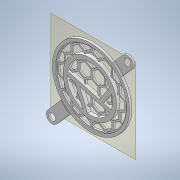
# Autodesk Inventor part: Rear Left Fan Cover
Saved by Autodesk Inventor 2020 (Build 240168000, 168)
## iProperties
Created: 2019-11-19
Part Number: Rear Left Fan Cover
Material: Generic
Document SubType Name: Modeling
Designer: pepd9
Density: 1 g/cm^3
Appearance: Default
Author: pepd9
Autodesk Inventor part; units mm, degrees
ref_plane "YZ Plane" through (0, 0, 0) normal (1, 0, 0) x (0, 1, 0)
ref_plane "XZ Plane" through (0, 0, 0) normal (0, 1, 0) x (-1, 0, 0)
ref_plane "XY Plane" through (0, 0, 0) normal (0, 0, 1) x (1, 0, 0)
sketch "Sketch1" plane through (0, 0, 0) normal (0, 0, 1) x (1, 0, 0)
  circle A0 centre (0, 0) radius 17.5
  circle A1 centre (0, 0) radius 19.5
  dimension "d0" = 35
  dimension "d1" = 2
  constraints: 2 centre point, 1 coincident
  measures "d0" diameter of A0
  measures "d1" radial gap between concentric circles of A0 A1
extrude "Extrusion1" add sketch "Sketch1" along normal blind 0.8
ref_plane "Work Plane1" through (0, 0, 0) normal (0, 0, 1) x (1, 0, 0)
sketch "Sketch2" plane through (0, 0, 0) normal (0, 0, 1) x (1, 0, 0)
  line L0 (0, 3.4641) -> (3, 1.7321)
  line L1 (3, 1.7321) -> (3, -1.7321)
  line L2 (3, -1.7321) -> (0, -3.4641)
  line L3 (0, -3.4641) -> (-3, -1.7321)
  line L4 (-3, -1.7321) -> (-3, 1.7321)
  line L5 (-3, 1.7321) -> (0, 3.4641)
  line L6 (0, 4.3879) -> (3.8, 2.1939)
  line L7 (3.8, 2.1939) -> (3.8, -2.1939)
  line L8 (3.8, -2.1939) -> (0, -4.3879)
  line L9 (0, -4.3879) -> (-3.8, -2.1939)
  line L10 (-3.8, -2.1939) -> (-3.8, 2.1939)
  line L11 (-3.8, 2.1939) -> (0, 4.3879)
  line L12 (26.5453, -9.9641) -> (29.5453, -11.6962)
  line L13 (29.5453, -11.6962) -> (29.5453, -15.1603)
  line L14 (29.5453, -15.1603) -> (26.5453, -16.8923)
  line L15 (26.5453, -16.8923) -> (23.5453, -15.1603)
  line L16 (23.5453, -15.1603) -> (23.5453, -11.6962)
  line L17 (23.5453, -11.6962) -> (26.5453, -9.9641)
  line L18 (26.5453, -9.0403) -> (30.3453, -11.2343)
  line L19 (30.3453, -11.2343) -> (30.3453, -15.6221)
  line L20 (30.3453, -15.6221) -> (26.5453, -17.8161)
  line L21 (26.5453, -17.8161) -> (22.7453, -15.6221)
  line L22 (22.7453, -15.6221) -> (22.7453, -11.2343)
  line L23 (22.7453, -11.2343) -> (26.5453, -9.0403)
  line L24 (-6.8, 3.4641) -> (-3.8, 1.7321)
  line L25 (-3.8, 1.7321) -> (-3.8, -1.7321)
  line L26 (-3.8, -1.7321) -> (-6.8, -3.4641)
  line L27 (-6.8, -3.4641) -> (-9.8, -1.7321)
  line L28 (-9.8, -1.7321) -> (-9.8, 1.7321)
  line L29 (-9.8, 1.7321) -> (-6.8, 3.4641)
  line L30 (-6.8, 4.3879) -> (-3, 2.1939)
  line L31 (-3, 2.1939) -> (-3, -2.1939)
  line L32 (-3, -2.1939) -> (-6.8, -4.3879)
  line L33 (-6.8, -4.3879) -> (-10.6, -2.1939)
  line L34 (-10.6, -2.1939) -> (-10.6, 2.1939)
  line L35 (-10.6, 2.1939) -> (-6.8, 4.3879)
  line L36 (-13.6, 3.4641) -> (-10.6, 1.7321)
  line L37 (-10.6, 1.7321) -> (-10.6, -1.7321)
  line L38 (-10.6, -1.7321) -> (-13.6, -3.4641)
  line L39 (-13.6, -3.4641) -> (-16.6, -1.7321)
  line L40 (-16.6, -1.7321) -> (-16.6, 1.7321)
  line L41 (-16.6, 1.7321) -> (-13.6, 3.4641)
  line L42 (-13.6, 4.3879) -> (-9.8, 2.1939)
  line L43 (-9.8, 2.1939) -> (-9.8, -2.1939)
  line L44 (-9.8, -2.1939) -> (-13.6, -4.3879)
  line L45 (-13.6, -4.3879) -> (-17.4, -2.1939)
  line L46 (-17.4, -2.1939) -> (-17.4, 2.1939)
  line L47 (-17.4, 2.1939) -> (-13.6, 4.3879)
  line L48 (-20.4, 3.4641) -> (-17.4, 1.7321)
  line L49 (-17.4, 1.7321) -> (-17.4, -1.7321)
  line L50 (-17.4, -1.7321) -> (-20.4, -3.4641)
  line L51 (-20.4, -3.4641) -> (-23.4, -1.7321)
  line L52 (-23.4, -1.7321) -> (-23.4, 1.7321)
  line L53 (-23.4, 1.7321) -> (-20.4, 3.4641)
  line L54 (-20.4, 4.3879) -> (-16.6, 2.1939)
  line L55 (-16.6, 2.1939) -> (-16.6, -2.1939)
  line L56 (-16.6, -2.1939) -> (-20.4, -4.3879)
  line L57 (-20.4, -4.3879) -> (-24.2, -2.1939)
  line L58 (-24.2, -2.1939) -> (-24.2, 2.1939)
  line L59 (-24.2, 2.1939) -> (-20.4, 4.3879)
  line L60 (6.8, 3.4641) -> (9.8, 1.7321)
  line L61 (9.8, 1.7321) -> (9.8, -1.7321)
  line L62 (9.8, -1.7321) -> (6.8, -3.4641)
  line L63 (6.8, -3.4641) -> (3.8, -1.7321)
  line L64 (3.8, -1.7321) -> (3.8, 1.7321)
  line L65 (3.8, 1.7321) -> (6.8, 3.4641)
  line L66 (6.8, 4.3879) -> (10.6, 2.1939)
  line L67 (10.6, 2.1939) -> (10.6, -2.1939)
  line L68 (10.6, -2.1939) -> (6.8, -4.3879)
  line L69 (6.8, -4.3879) -> (3, -2.1939)
  line L70 (3, -2.1939) -> (3, 2.1939)
  line L71 (3, 2.1939) -> (6.8, 4.3879)
  line L72 (13.6, 3.4641) -> (16.6, 1.7321)
  line L73 (16.6, 1.7321) -> (16.6, -1.7321)
  line L74 (16.6, -1.7321) -> (13.6, -3.4641)
  line L75 (13.6, -3.4641) -> (10.6, -1.7321)
  line L76 (10.6, -1.7321) -> (10.6, 1.7321)
  line L77 (10.6, 1.7321) -> (13.6, 3.4641)
  line L78 (13.6, 4.3879) -> (17.4, 2.1939)
  line L79 (17.4, 2.1939) -> (17.4, -2.1939)
  line L80 (17.4, -2.1939) -> (13.6, -4.3879)
  line L81 (13.6, -4.3879) -> (9.8, -2.1939)
  line L82 (9.8, -2.1939) -> (9.8, 2.1939)
  line L83 (9.8, 2.1939) -> (13.6, 4.3879)
  line L84 (17.4, -2.1939) -> (17.4, 2.1939)
  line L85 (10.2, 9.3531) -> (13.2, 7.621)
  line L86 (13.2, 7.621) -> (13.2, 4.1569)
  line L87 (7.2, 4.1569) -> (7.2, 7.621)
  line L88 (7.2, 7.621) -> (10.2, 9.3531)
  line L89 (10.2, 10.2768) -> (14, 8.0829)
  line L90 (14, 8.0829) -> (14, 4.1569)
  line L91 (6.4, 4.1569) -> (6.4, 8.0829)
  line L92 (6.4, 8.0829) -> (10.2, 10.2768)
  line L93 (3.4, 9.3531) -> (6.4, 7.621)
  line L94 (0.4, 4.1569) -> (0.4, 7.621)
  line L95 (0.4, 7.621) -> (3.4, 9.3531)
  line L96 (3.4, 10.2768) -> (6.8, 8.3138)
  line L97 (-0.4, 4.1569) -> (-0.4, 8.0829)
  line L98 (-0.4, 8.0829) -> (3.4, 10.2768)
  line L99 (-3.4, 9.3531) -> (-0.4, 7.621)
  line L100 (-6.4, 4.1569) -> (-6.4, 7.621)
  line L101 (-6.4, 7.621) -> (-3.4, 9.3531)
  line L102 (-3.4, 10.2768) -> (0, 8.3138)
  line L103 (-7.2, 4.1569) -> (-7.2, 8.0829)
  line L104 (-7.2, 8.0829) -> (-3.4, 10.2768)
  line L105 (-10.2, 9.3531) -> (-7.2, 7.621)
  line L106 (-13.2, 4.1569) -> (-13.2, 7.621)
  line L107 (-13.2, 7.621) -> (-10.2, 9.3531)
  line L108 (-10.2, 10.2768) -> (-6.8, 8.3138)
  line L109 (-14, 4.1569) -> (-14, 8.0829)
  line L110 (-14, 8.0829) -> (-10.2, 10.2768)
  line L111 (-17, 9.3531) -> (-14, 7.621)
  line L112 (-20, 4.1569) -> (-20, 7.621)
  line L113 (-20, 7.621) -> (-17, 9.3531)
  line L114 (-17, 10.2768) -> (-13.6, 8.3138)
  line L115 (-20.8, 3.695) -> (-20.8, 8.0829)
  line L116 (-20.8, 8.0829) -> (-17, 10.2768)
  line L117 (13.6, 8.3138) -> (17, 10.2768)
  line L118 (14, 7.621) -> (17, 9.3531)
  line L119 (17, 10.2768) -> (20.8, 8.0829)
  line L120 (17, 9.3531) -> (20, 7.621)
  line L121 (13.6, 15.242) -> (16.6, 13.51)
  line L122 (16.6, 13.51) -> (16.6, 10.0459)
  line L123 (10.6, 10.0459) -> (10.6, 13.51)
  line L124 (10.6, 13.51) -> (13.6, 15.242)
  line L125 (13.6, 16.1658) -> (17.4, 13.9719)
  line L126 (17.4, 13.9719) -> (17.4, 9.584)
  line L127 (9.8, 10.0459) -> (9.8, 13.9719)
  line L128 (9.8, 13.9719) -> (13.6, 16.1658)
  line L129 (6.8, 15.242) -> (9.8, 13.51)
  line L130 (3.8, 10.0459) -> (3.8, 13.51)
  line L131 (3.8, 13.51) -> (6.8, 15.242)
  line L132 (6.8, 16.1658) -> (10.6, 13.9719)
  line L133 (3, 10.0459) -> (3, 13.9719)
  line L134 (3, 13.9719) -> (6.8, 16.1658)
  line L135 (0, 15.242) -> (3, 13.51)
  line L136 (-3, 10.0459) -> (-3, 13.51)
  line L137 (-3, 13.51) -> (0, 15.242)
  line L138 (0, 16.1658) -> (3.4, 14.2028)
  line L139 (-3.8, 10.0459) -> (-3.8, 13.9719)
  line L140 (-3.8, 13.9719) -> (0, 16.1658)
  line L141 (-6.8, 15.242) -> (-3.8, 13.51)
  line L142 (-9.8, 10.0459) -> (-9.8, 13.51)
  line L143 (-9.8, 13.51) -> (-6.8, 15.242)
  line L144 (-6.8, 16.1658) -> (-3.4, 14.2028)
  line L145 (-10.6, 10.0459) -> (-10.6, 13.9719)
  line L146 (-10.6, 13.9719) -> (-6.8, 16.1658)
  line L147 (-13.6, 15.242) -> (-10.6, 13.51)
  line L148 (-16.6, 10.0459) -> (-16.6, 13.51)
  line L149 (-16.6, 13.51) -> (-13.6, 15.242)
  line L150 (-13.6, 16.1658) -> (-10.2, 14.2028)
  line L151 (-17.4, 9.584) -> (-17.4, 13.9719)
  line L152 (-17.4, 13.9719) -> (-13.6, 16.1658)
  line L153 (10.2, 21.131) -> (13.2, 19.399)
  line L154 (13.2, 19.399) -> (13.2, 15.9349)
  line L155 (7.2, 15.9349) -> (7.2, 19.399)
  line L156 (7.2, 19.399) -> (10.2, 21.131)
  line L157 (10.2, 22.0548) -> (14, 19.8608)
  line L158 (14, 19.8608) -> (14, 15.473)
  line L159 (6.4, 15.473) -> (6.4, 19.8608)
  line L160 (6.4, 19.8608) -> (10.2, 22.0548)
  line L161 (3.4, 21.131) -> (6.4, 19.399)
  line L162 (0.4, 15.9349) -> (0.4, 19.399)
  line L163 (0.4, 19.399) -> (3.4, 21.131)
  line L164 (3.4, 22.0548) -> (7.2, 19.8608)
  line L165 (-0.4, 15.473) -> (-0.4, 19.8608)
  line L166 (-0.4, 19.8608) -> (3.4, 22.0548)
  line L167 (-3.4, 21.131) -> (-0.4, 19.399)
  line L168 (-6.4, 15.9349) -> (-6.4, 19.399)
  line L169 (-6.4, 19.399) -> (-3.4, 21.131)
  line L170 (-3.4, 22.0548) -> (0.4, 19.8608)
  line L171 (-7.2, 15.473) -> (-7.2, 19.8608)
  line L172 (-7.2, 19.8608) -> (-3.4, 22.0548)
  line L173 (20.4, -7.3901) -> (17.4, -9.1221)
  line L174 (17.4, -9.1221) -> (14.4, -7.3901)
  line L175 (14.4, -7.3901) -> (14.4, -3.926)
  line L176 (21.2, -7.852) -> (17.4, -10.0459)
  line L177 (17.4, -10.0459) -> (13.6, -7.852)
  line L178 (13.6, -7.852) -> (13.6, -3.4641)
  line L179 (13.6, -7.3901) -> (10.2, -9.3531)
  line L180 (10.2, -9.3531) -> (7.2, -7.621)
  line L181 (7.2, -7.621) -> (7.2, -4.1569)
  line L182 (14, -8.0829) -> (10.2, -10.2768)
  line L183 (10.2, -10.2768) -> (6.4, -8.0829)
  line L184 (6.4, -8.0829) -> (6.4, -4.1569)
  line L185 (6.4, -7.621) -> (3.4, -9.3531)
  line L186 (3.4, -9.3531) -> (0.4, -7.621)
  line L187 (0.4, -7.621) -> (0.4, -4.1569)
  line L188 (6.8, -8.3138) -> (3.4, -10.2768)
  line L189 (3.4, -10.2768) -> (-0.4, -8.0829)
  line L190 (-0.4, -8.0829) -> (-0.4, -3.695)
  line L191 (-0.4, -7.621) -> (-3.4, -9.3531)
  line L192 (-3.4, -9.3531) -> (-6.4, -7.621)
  line L193 (-6.4, -7.621) -> (-6.4, -4.1569)
  line L194 (0, -8.3138) -> (-3.4, -10.2768)
  line L195 (-3.4, -10.2768) -> (-7.2, -8.0829)
  line L196 (-7.2, -8.0829) -> (-7.2, -3.695)
  line L197 (-7.2, -7.621) -> (-10.2, -9.3531)
  line L198 (-10.2, -9.3531) -> (-13.2, -7.621)
  line L199 (-13.2, -7.621) -> (-13.2, -4.1569)
  line L200 (-6.8, -8.3138) -> (-10.2, -10.2768)
  line L201 (-10.2, -10.2768) -> (-14, -8.0829)
  line L202 (-14, -8.0829) -> (-14, -3.695)
  line L203 (-14, -7.621) -> (-17, -9.3531)
  line L204 (-17, -9.3531) -> (-20, -7.621)
  line L205 (-20, -7.621) -> (-20, -4.1569)
  line L206 (-13.6, -8.3138) -> (-17, -10.2768)
  line L207 (-17, -10.2768) -> (-20.8, -8.0829)
  line L208 (-20.8, -8.0829) -> (-20.8, -3.695)
  line L209 (17, -9.815) -> (17, -13.2791)
  line L210 (17, -13.2791) -> (14, -15.0111)
  line L211 (14, -15.0111) -> (11, -13.2791)
  line L212 (11, -13.2791) -> (11, -9.815)
  line L213 (17.8, -9.3531) -> (17.8, -13.7409)
  line L214 (17.8, -13.7409) -> (14, -15.9349)
  line L215 (14, -15.9349) -> (10.2, -13.7409)
  line L216 (10.2, -13.7409) -> (10.2, -9.3531)
  line L217 (10.2, -13.2791) -> (6.8, -15.242)
  line L218 (6.8, -15.242) -> (3.8, -13.51)
  line L219 (3.8, -13.51) -> (3.8, -10.0459)
  line L220 (10.6, -13.9719) -> (6.8, -16.1658)
  line L221 (6.8, -16.1658) -> (3, -13.9719)
  line L222 (3, -13.9719) -> (3, -9.584)
  line L223 (3, -13.51) -> (0, -15.242)
  line L224 (0, -15.242) -> (-3, -13.51)
  line L225 (-3, -13.51) -> (-3, -10.0459)
  line L226 (3.8, -13.9719) -> (0, -16.1658)
  line L227 (0, -16.1658) -> (-3.8, -13.9719)
  line L228 (-3.8, -13.9719) -> (-3.8, -9.584)
  line L229 (-3.8, -13.51) -> (-6.8, -15.242)
  line L230 (-6.8, -15.242) -> (-9.8, -13.51)
  line L231 (-9.8, -13.51) -> (-9.8, -10.0459)
  line L232 (-3, -13.9719) -> (-6.8, -16.1658)
  line L233 (-6.8, -16.1658) -> (-10.6, -13.9719)
  line L234 (-10.6, -13.9719) -> (-10.6, -9.584)
  line L235 (-10.6, -13.51) -> (-13.6, -15.242)
  line L236 (-13.6, -15.242) -> (-16.6, -13.51)
  line L237 (-16.6, -13.51) -> (-16.6, -10.0459)
  line L238 (-9.8, -13.9719) -> (-13.6, -16.1658)
  line L239 (-13.6, -16.1658) -> (-17.4, -13.9719)
  line L240 (-17.4, -13.9719) -> (-17.4, -9.584)
  line L241 (13.6, -15.7039) -> (13.6, -19.168)
  line L242 (13.6, -19.168) -> (10.6, -20.9001)
  line L243 (10.6, -20.9001) -> (7.6, -19.168)
  line L244 (7.6, -19.168) -> (7.6, -15.7039)
  line L245 (14.4, -15.242) -> (14.4, -19.6299)
  line L246 (14.4, -19.6299) -> (10.6, -21.8238)
  line L247 (10.6, -21.8238) -> (6.8, -19.6299)
  line L248 (6.8, -19.6299) -> (6.8, -15.242)
  line L249 (6.4, -19.399) -> (3.4, -21.131)
  line L250 (3.4, -21.131) -> (0.4, -19.399)
  line L251 (0.4, -19.399) -> (0.4, -15.9349)
  line L252 (7.2, -19.8608) -> (3.4, -22.0548)
  line L253 (3.4, -22.0548) -> (-0.4, -19.8608)
  line L254 (-0.4, -19.8608) -> (-0.4, -15.473)
  line L255 (-0.4, -19.399) -> (-3.4, -21.131)
  line L256 (-3.4, -21.131) -> (-6.4, -19.399)
  line L257 (-6.4, -19.399) -> (-6.4, -15.9349)
  line L258 (0.4, -19.8608) -> (-3.4, -22.0548)
  line L259 (-3.4, -22.0548) -> (-7.2, -19.8608)
  line L260 (-7.2, -19.8608) -> (-7.2, -15.473)
  line L261 (-7.2, -19.399) -> (-10.2, -21.131)
  line L262 (-10.2, -21.131) -> (-13.2, -19.399)
  line L263 (-13.2, -19.399) -> (-13.2, -15.9349)
  line L264 (-6.4, -19.8608) -> (-10.2, -22.0548)
  line L265 (-10.2, -22.0548) -> (-14, -19.8608)
  line L266 (-14, -19.8608) -> (-14, -15.473)
  circle A0 centre (0, 0) radius 17.5 projected
  line L267 (20.4, 3.4641) -> (23.4, 1.7321)
  line L268 (23.4, 1.7321) -> (23.4, -1.7321)
  line L269 (23.4, -1.7321) -> (20.4, -3.4641)
  line L270 (20.4, -3.4641) -> (17.4, -1.7321)
  line L271 (17.4, -1.7321) -> (17.4, 1.7321)
  line L272 (17.4, 1.7321) -> (20.4, 3.4641)
  line L273 (20.4, 4.3879) -> (24.2, 2.1939)
  line L274 (24.2, 2.1939) -> (24.2, -2.1939)
  line L275 (24.2, -2.1939) -> (20.4, -4.3879)
  line L276 (20.4, -4.3879) -> (16.6, -2.1939)
  line L277 (16.6, -2.1939) -> (16.6, 2.1939)
  line L278 (16.6, 2.1939) -> (20.4, 4.3879)
  point P0 (26.5453, -13.4282)
  point P1 (-3.8, 1.7321)
  point P2 (-6.8, 0)
  point P3 (-10.6, 1.7321)
  point P4 (-13.6, 0)
  point P5 (-17.4, 1.7321)
  point P6 (-20.4, 0)
  point P7 (-24.2, 1.7321)
  point P8 (30.3453, -11.6962)
  point P9 (22.7453, -11.6962)
  point P10 (6.8, 0)
  point P11 (10.6, 1.7321)
  point P12 (3, 1.7321)
  point P13 (13.6, 0)
  point P14 (21.2, 0)
  point P15 (-17, 2.4249)
  point P16 (-10.2, 2.4249)
  point P17 (-3.4, 2.4249)
  point P18 (3.4, 2.4249)
  point P19 (10.2, 2.4249)
  point P20 (10.2, -2.4249)
  point P21 (3.4, -2.4249)
  point P22 (-3.4, -2.4249)
  point P23 (-10.2, -2.4249)
  point P24 (-17, -2.4249)
  point P25 (10.2, 5.889)
  point P26 (14, 7.621)
  point P27 (6.4, 7.621)
  point P28 (3.4, 5.889)
  point P29 (-0.4, 7.621)
  point P30 (-3.4, 5.889)
  point P31 (-7.2, 7.621)
  point P32 (-10.2, 5.889)
  point P33 (-14, 7.621)
  point P34 (-17, 5.889)
  point P35 (-20.8, 7.621)
  point P36 (13.6, 8.3138)
  point P37 (-6.8, 8.3138)
  point P38 (13.6, 11.7779)
  point P39 (17.4, 13.51)
  point P40 (9.8, 13.51)
  point P41 (6.8, 11.7779)
  point P42 (3, 13.51)
  point P43 (0, 11.7779)
  point P44 (-3.8, 13.51)
  point P45 (-6.8, 11.7779)
  point P46 (-10.6, 13.51)
  point P47 (-13.6, 11.7779)
  point P48 (-17.4, 13.51)
  point P49 (10.2, 14.2028)
  point P50 (14, 19.399)
  point P51 (6.4, 19.399)
  point P52 (-0.4, 19.399)
  point P53 (-7.2, 19.399)
  point P54 (17.4, -5.658)
  point P55 (10.2, -5.889)
  point P56 (3.4, -5.889)
  point P57 (-0.4, -4.1569)
  point P58 (-3.4, -5.889)
  point P59 (-7.2, -4.1569)
  point P60 (-10.2, -5.889)
  point P61 (-14, -4.1569)
  point P62 (-17, -5.889)
  point P63 (-20.8, -4.1569)
  point P64 (14, -8.0829)
  point P65 (0, -8.3138)
  point P66 (-3.4, -14.2028)
  point P67 (3.4, -14.2028)
  point P68 (-10.2, -14.2028)
  point P69 (10.6, -13.9719)
  point P70 (10.6, -17.436)
  point P71 (3.4, -17.6669)
  point P72 (-3.4, -17.6669)
  point P73 (-10.2, -17.6669)
  point P74 (20.4, 0)
  point P75 (24.2, 1.7321)
  point P76 (16.6, 1.7321)
  point P77 (-0.4, 7.621)
  point P78 (-0.4, -4.1569)
  point P79 (-3.8, -1.7321)
  point P80 (-10.2, 2.4249)
  point P81 (-7.2, -4.1569)
  point P82 (3.4, 2.4249)
  point P83 (6.4, 7.621)
  point P84 (-17.3056, 2.6013)
  point P85 (-17.4, 1.8682)
  point P86 (-17.4, -1.7321)
  point P87 (-17.4133, -1.7397)
  point P88 (-17.3056, -2.6013)
  point P89 (-14, -4.1569)
  point P90 (-15.3515, -8.4013)
  point P91 (-14.9515, -9.0941)
  point P92 (-10.6, -10.0459)
  point P93 (-10.9056, -13.6864)
  point P94 (-10.3179, -14.1348)
  point P95 (-7.2, -15.9349)
  point P96 (-7.2, -15.9502)
  point P97 (-6.4, -16.2877)
  point P98 (-0.4, -15.9349)
  point P99 (-0.4, -17.4954)
  point P100 (0.4, -17.4954)
  point P101 (6.7589, -16.1421)
  point P102 (7.6, -15.7636)
  point P103 (10.3179, -14.1348)
  point P104 (11.2368, -13.4158)
  point P105 (15.1554, -8.75)
  point P106 (15.5396, -8.048)
  point P107 (17, -2.4249)
  point P108 (17.3056, -2.6013)
  point P109 (17.4, -1.8682)
  point P110 (17.4, 1.8682)
  point P111 (17.3056, 2.6013)
  point P112 (17, 2.4249)
  point P113 (15.3515, 8.4013)
  point P114 (14.9515, 9.0941)
  point P115 (10.9056, 13.6864)
  point P116 (10.3179, 14.1348)
  point P117 (7.0821, 16.0029)
  point P118 (6.4, 16.2877)
  point P119 (6.4, 15.9349)
  point P120 (0.4, 17.4954)
  point P121 (-0.4, 17.4954)
  point P122 (-0.4, 15.9349)
  point P123 (-6.4, 15.9349)
  point P124 (-6.4, 16.2877)
  point P125 (-7.0821, 16.0029)
  point P126 (-10.2133, 14.2105)
  point P127 (-10.9056, 13.6864)
  point P128 (-14.9515, 9.0941)
  point P129 (-15.3515, 8.4013)
  point P130 (3, -10.0459)
  point P131 (-3.8, -10.0459)
  point P132 (-9.8, 10.0459)
  point P133 (-10.6, -1.7321)
  dimension "d5" = 6
  dimension "d6" = 0.8
  dimension "d8" = 6
  dimension "d9" = 0.8
  dimension "d10" = 0.8
  dimension "d11" = 6
  dimension "d12" = 0.8
  dimension "d13" = 0.8
  dimension "d14" = 6
  dimension "d15" = 0.8
  dimension "d16" = 0.8
  dimension "d17" = 6
  dimension "d18" = 0.8
  dimension "d19" = 0.8
  dimension "d20" = 6
  dimension "d21" = 0.8
  dimension "d22" = 6
  dimension "d23" = 0.8
  dimension "d26" = 6
  dimension "d27" = 0.8
  dimension "d28" = 0.8
  dimension "d29" = 0.8
  dimension "d30" = 0.8
  dimension "d31" = 0.8
  dimension "d33" = 0.8
  dimension "d34" = 6
  dimension "d35" = 0.8
  dimension "d36" = 0.8
  dimension "d37" = 0.8
  dimension "d38" = 0.8
  dimension "d39" = 0.8
  dimension "d40" = 6
  dimension "d41" = 0.8
  dimension "d42" = 0.8
  dimension "d43" = 0.8
  dimension "d45" = 6
  dimension "d46" = 6
  dimension "d47" = 6
  dimension "d48" = 0.8
  constraints: 558 end point, 79 point on line, 33 horizontal alignment, 15 coincident, 177 other
  measures "d5" distance between parallel lines of L1 L4
  measures "d6" distance between parallel lines of L5 L11
  measures "d8" distance between parallel lines of L13 L16
  measures "d9" distance between parallel lines of L17 L23
  measures "d10" distance of L4.end point (-3.8, 1.732)
  measures "d11" distance between parallel lines of L25 L28
  measures "d12" distance between parallel lines of L29 L35
  measures "d13" distance of L28.end point (-10.6, 1.732)
  measures "d14" distance between parallel lines of L37 L40
  measures "d15" distance between parallel lines of L41 L47
  measures "d16" distance of L40.end point (-17.4, 1.732)
  measures "d17" distance between parallel lines of L49 L52
  measures "d18" distance between parallel lines of L53 L59
  measures "d19" distance of L52.end point (-24.2, 1.732)
  measures "d20" distance between parallel lines of L61 L64
  measures "d21" distance between parallel lines of L65 L71
  measures "d22" distance between parallel lines of L73 L76
  measures "d23" distance between parallel lines of L77 L83
  measures "d26" distance between parallel lines of L86 L87
  measures "d27" distance between parallel lines of L88 L92
  measures "d28" distance between parallel lines of L95 L98
  measures "d29" distance between parallel lines of L101 L104
  measures "d30" distance between parallel lines of L107 L110
  measures "d31" distance between parallel lines of L113 L116
  measures "d33" distance between parallel lines of L118 L117
  measures "d34" distance between parallel lines of L122 L123
  measures "d35" distance between parallel lines of L124 L128
  measures "d36" distance between parallel lines of L131 L134
  measures "d37" distance between parallel lines of L137 L140
  measures "d38" distance between parallel lines of L143 L146
  measures "d39" distance between parallel lines of L149 L152
  measures "d40" distance between parallel lines of L154 L155
  measures "d41" distance between parallel lines of L156 L160
  measures "d42" distance between parallel lines of L163 L166
  measures "d43" distance between parallel lines of L169 L172
  measures "d45" distance between parallel lines of L209 L212
  measures "d46" distance between parallel lines of L241 L244
  measures "d47" distance between parallel lines of L268 L271
  measures "d48" distance between parallel lines of L272 L278
extrude "Extrusion2" add sketch "Sketch2" along normal blind 0.8 contours L5 L31 L30 L11 L6 L71 L70 L0 | L70 L71 L6 L7 L8 L69 L1 | L4 L31 L32 L9 L10 L11 L30 | L70 L69 L8 L9 L32 L31 L3 L2 | L71 L66 L83 L82 L60 L65 L7 L6 | L11 L10 L24 L29 L43 L42 L35 L30 | L8 L7 L63 L62 L82 L81 L68 L69 | L6 L11 L97 L98 L96 L92 L91 L93 L95 L94 | L91 L92 L89 L90 L78 L83 L86 L85 L88 L87 L66 L71 | L32 L33 L44 L43 L27 L26 L10 L9 | L30 L35 L103 L104 L102 L98 L97 L99 L101 L100 | L187 L186 L185 L184 L183 L188 L189 L190 L9 L8 | L69 L68 L181 L180 L216 L183 L184 | L193 L192 L191 L190 L189 L194 L195 L196 L33 L32 | L82 L83 L66 L67 L68 L81 L61 | L83 L78 L278 L277 L72 L77 L67 L66 | L28 L43 L44 L33 L34 L35 L42 | L35 L34 L36 L41 L55 L54 L47 L42 | L105 L107 L106 L42 L47 L109 L110 L108 L104 L103 | L68 L67 L75 L178 L81 | L127 L128 L132 A0 L124 L123 L89 L92 | L96 L98 L133 L134 A0 L132 L128 L127 L129 L131 L130 | L44 L45 L56 L55 L39 L38 L34 L33 | L196 L195 L200 L201 L202 L45 L44 L199 L198 L197 | L102 L104 L139 L140 L138 L134 L133 L135 L137 L136 | L178 L74 L277 L276 L80 | L80 L175 L174 A0 L177 L178 | L179 L178 L177 L182 L216 | L182 L212 L211 A0 L215 L216 | L219 L218 L248 A0 L221 L222 L189 L188 | L225 L224 L223 L222 L221 L226 L227 L228 L195 L194 | L216 L215 A0 L220 L248 L217 | L108 L110 L145 A0 L146 L144 L140 L139 L141 L143 L142 | L276 L277 L73 L278 L78 A0 L79 L80 | L80 A0 L276 | L278 A0 L78 | L90 L89 L117 A0 L118 | L231 L230 L229 L228 L227 L232 A0 L233 L234 L201 L200 | L40 L55 L56 L45 A0 L46 L47 L54 | L47 A0 L54 | L111 A0 L114 L110 L109 | L56 A0 L45 | L202 L201 L206 A0 L203 | L159 A0 L134 | L138 L140 L165 A0 L162 | L220 L244 A0 | L251 A0 L254 L227 L226 | L147 A0 L145 | A0 L50 L46 | L234 A0 L235 | L144 A0 L168 | L257 A0 L232 | A0 L150 L146 | A0 L260 L233 picked at (7.3126, -15.8773)
sketch "Sketch3" plane through (0, 0, 0.8) normal (0, 0, 1) x (1, 0, 0)
  circle A0 centre (0, 0) radius 18
  circle A1 centre (0, 0) radius 19.5
  dimension "d51" = 36
  dimension "d52" = 39
  constraints: 2 centre point, 2 coincident
  measures "d51" diameter of A0
  measures "d52" diameter of A1
extrude "Extrusion3" add sketch "Sketch3" along normal blind 0.4
sketch "Sketch4" plane through (0, 0, 0) normal (0, 0, 1) x (1, 0, 0)
  circle A0 centre (0, 0) radius 13.5
  circle A1 centre (0, 0) radius 11.5
  line L0 (-11.3248, 2) -> (10.8075, -3.9303)
  line L1 (-11.5, -0.0236) -> (9.9475, -5.7704)
  line L2 (0, 0) -> (-14.9, 0) construction
  line L3 (4.8066, -2.3224) -> (10.1794, 5.3507)
  line L4 (-7.4581, -1.1066) -> (-3.4762, -10.962)
  line L5 (-5.0391, -1.7548) -> (-1.124, -11.4449)
  line L6 (6.8624, -2.8732) -> (11.0659, 3.1299)
  dimension "d56" = 23
  dimension "d55" = 27
  dimension "d57" = 2
  dimension "d58" = 2
  dimension "d59" = 15
  dimension "d60" = 2
  dimension "d61" = 2
  dimension "d62" = 112
  dimension "d63" = 125
  constraints: 14 end point, 4 point on line, 3 parallel, 2 coincident, 1 centre point, 1 horizontal, 10 other
  measures "d55" diameter of A0
  measures "d57" distance between parallel lines of L1 L0
  measures "d58" vertical distance of point (0, 0) L0.start
  measures "d59" angle of L1 L2
  measures "d60" distance between parallel lines of L4 L5
  measures "d61" distance between parallel lines of L3 L6
  measures "d62" angle of L2 L4
  measures "d63" angle of L2 L6
extrude "Extrusion4" add sketch "Sketch4" along normal blind 1.8 contours A0 | L6 L0 L3 A1 | A1 L1 L0 | A1 L4 L1 L5
sketch "Sketch5" plane through (0, 0, 0) normal (0, 0, 1) x (1, 0, 0)
  circle A0 centre (18, 20) radius 2.55 construction
  circle A1 centre (-20, -23) radius 2.55 construction
  circle A2 centre (0, 0) radius 19.5 projected
  circle A3 centre (-20, -23) radius 1.7
  circle A4 centre (-20, -23) radius 3
  circle A5 centre (18, 20) radius 3
  circle A6 centre (18, 20) radius 1.7
  line L0 (-17.5566, -24.7407) -> (20.4434, 18.2593)
  line L1 (15.5566, 21.7407) -> (-22.4434, -21.2593)
  point P0 (-15.6171, -11.6772)
  point P1 (-11.2687, -15.9143)
  point P2 (11.3598, 15.8495)
  point P3 (15.6871, 11.5829)
  point P4 (10.7319, 16.2811)
  point P5 (15.1532, 12.2731)
  point P6 (20.028, 17.7893)
  point P7 (-14.8376, -12.6528)
  point P8 (-22.028, -20.7893)
  point P9 (-10.3163, -16.5476)
  dimension "d66" = 3.4
  dimension "d67" = 6
  dimension "d68" = 6
  dimension "d70" = 3.4
  constraints: 8 point on circle, 4 centre point, 4 coincident, 4 end point
  measures "d66" diameter of A3
  measures "d67" diameter of A4
  measures "d68" diameter of A5
  measures "d70" diameter of A6
extrude "Extrusion5" add sketch "Sketch5" along normal blind 0.8 contours A2 L1 A5 L0 | L0 A4 L1 A2 | L0 A5 | A5 L0 | A4 L1 | L1 A4
fillet "Fillet1" radius 2 2 edges at (13.0968, 14.4473, 0.8) (-12.7268, -14.7742, 0.8)
fillet "Fillet2" radius 4 4 edges at (-10.3163, -16.5476, 0.6) (-14.8376, -12.6528, 0.6) (15.1532, 12.2731, 0.6) (10.7319, 16.2811, 0.6)
body "Solid1"
